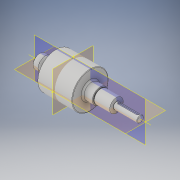
# Autodesk Inventor part: vratilo
Saved by Autodesk Inventor 2018 (Build 220112000, 112)
## iProperties
Created: 2018-05-05
Part Number: vratilo
Material: Generic
Document SubType Name: Modeling
Designer: Kristijan
Density: 1 g/cm^3
Appearance: Default
Author: Kristijan
Autodesk Inventor part; units mm, degrees
sketch "Sketch1" plane through (0, 0, 0) normal (1, 0, 0) x (0, 1, 0)
  circle A0 centre (0, 0) radius 60.5
  dimension "d0" = 121
  constraints: 1 centre point, 1 coincident
  measures "d0" diameter of A0
extrude "Extrusion1" add sketch "Sketch1" along normal mid plane 115
sketch "Sketch2" plane through (57.5, 0, 0) normal (1, 0, 0) x (0, 0, -1)
  circle A0 centre (0, 0) radius 26
  dimension "d3" = 52
  constraints: 1 centre point, 1 coincident
  measures "d3" diameter of A0
extrude "Extrusion2" add sketch "Sketch2" along normal blind 33
sketch "Sketch3" plane through (90.5, 0, 0) normal (1, 0, 0) x (0, 0, -1)
  circle A0 centre (0, 0) radius 22.5
  dimension "d6" = 45
  constraints: 1 centre point, 1 coincident
  measures "d6" diameter of A0
extrude "Extrusion3" add sketch "Sketch3" along normal blind 54
sketch "Sketch4" plane through (144.5, 0, 0) normal (1, 0, 0) x (0, 0, -1)
  circle A0 centre (0, 0) radius 11
  dimension "d9" = 22
  constraints: 1 centre point, 1 coincident
  measures "d9" diameter of A0
extrude "Extrusion4" add sketch "Sketch4" along normal blind 80
mirror "Mirror1" about plane through (0, 0, 0) normal (1, 0, 0) of "Extrusion2"
sketch "Sketch5" plane through (-90.5, 0, 0) normal (-1, 0, 0) x (0, 0, 1)
  circle A0 centre (0, 0) radius 22.5
  dimension "d12" = 45
  constraints: 1 centre point, 1 coincident
  measures "d12" diameter of A0
extrude "Extrusion5" add sketch "Sketch5" along normal blind 21
ref_plane "Work Plane1" through (144.5, 0, 11) normal (0, 0, 1) x (1, 0, 0)
sketch "Sketch6" plane through (144.5, 0, 11) normal (0, 0, 1) x (1, 0, 0)
  line L0 (9, 0) -> (71, 0) construction
  line L1 (9, -4) -> (71, -4)
  line L2 (71, 4) -> (9, 4)
  arc A0 (9, 4) -> (9, -4) centre (9, 0) ccw
  arc A1 (71, -4) -> (71, 4) centre (71, 0) ccw
  line L3 (80, -11) -> (80, 11) construction
  line L4 (-258.4, 0) -> (136.4, 0) construction
  line L5 (0, -22.5) -> (0, 22.5) construction
  point P0 (-144.5, 0)
  point P1 (40, 0)
  dimension "d15" = 62
  dimension "d16" = 8
  dimension "d18" = 5
  constraints: 8 end point, 4 point on circle, 4 tangent, 2 centre point, 1 collinear, 1 horizontal, 1 midpoint, 1 parallel
  measures "d15" distance of L0.start L0.end
  measures "d16" diameter of A1
  measures "d18" distance edge to line of A1 L3
extrude "Extrusion6" cut sketch "Sketch6" against normal blind 5
sketch "Sketch7" plane through (0, 0, 0) normal (0, 1, 0) x (-1, 0, 0)
  line L0 (-57.5, -26) -> (-90.5, -26) construction
  line L1 (-90.5, -26) -> (-90.5, -22.5) construction
  line L2 (-90.5, -22.5) -> (-144.5, -22.5) construction
  line L3 (-144.5, -22.5) -> (-144.5, -11) construction
  line L4 (-144.5, -11) -> (-224.5, -11) construction
  line L5 (-224.5, -11) -> (-224.5, 11) construction
  line L6 (-224.5, 11) -> (-219.5, 11) construction
  line L7 (-219.5, 11) -> (-219.5, 6) construction
  line L8 (-219.5, 6) -> (-149.5, 6) construction
  line L9 (-149.5, 6) -> (-149.5, 11) construction
  line L10 (-149.5, 11) -> (-144.5, 11) construction
  line L11 (-144.5, 11) -> (-144.5, 22.5) construction
  line L12 (-144.5, 22.5) -> (-90.5, 22.5) construction
  line L13 (-90.5, 22.5) -> (-90.5, 26) construction
  line L14 (-90.5, 26) -> (-57.5, 26) construction
  line L15 (-57.5, 26) -> (-57.5, 60.5) construction
  line L16 (-57.5, 60.5) -> (57.5, 60.5) construction
  line L17 (57.5, 60.5) -> (57.5, 26) construction
  line L18 (57.5, 26) -> (90.5, 26) construction
  line L19 (90.5, 26) -> (90.5, 22.5) construction
  line L20 (90.5, 22.5) -> (111.5, 22.5) construction
  line L21 (111.5, 22.5) -> (111.5, -22.5) construction
  line L22 (111.5, -22.5) -> (90.5, -22.5) construction
  line L23 (90.5, -22.5) -> (90.5, -26) construction
  line L24 (90.5, -26) -> (57.5, -26) construction
  line L25 (57.5, -26) -> (57.5, -60.5) construction
  line L26 (57.5, -60.5) -> (-57.5, -60.5) construction
  line L27 (-57.5, -60.5) -> (-57.5, -26) construction
  line L28 (-93, 15.4374) -> (-93, 22.5) construction
  line L29 (-90.5, 22.5) -> (-144.5, 22.5) construction
  line L30 (-93, 22.5) -> (-90.5, 22.5)
  line L31 (-90.5, 22.2) -> (-91.8804, 22.2)
  line L32 (-90.5, 26) -> (-90.5, -26) construction
  line L33 (-93, 22.5) -> (-91.8804, 22.2)
  line L34 (-90.5, 22.5) -> (-93, 22.5) construction
  line L35 (-90.5, 22.5) -> (-90.5, 22.2)
  line L36 (125.9, 0) -> (-198.9, 0) projected
  point P0 (0, 0)
  dimension "d21" = 2.5
  dimension "d24" = 0.3
  dimension "d25" = 15
  constraints: 12 end point, 3 point on line, 2 collinear, 2 horizontal, 1 vertical
  measures "d21" distance between parallel lines of L28 L13
  measures "d24" distance between parallel lines of L12 L31
  measures "d25" angle of L12 L33
revolve "Revolution1" cut sketch "Sketch7" angle 360 about axis through (-10, 0, 0) along (1, 0, 0)
mirror "Mirror2" about plane through (0, 0, 0) normal (1, 0, 0) of "Revolution1"
fillet "Fillet1" radius 0.6 1 edges at (90.5, 0, -22.2)
fillet "Fillet2" radius 0.6 1 edges at (91.8804, 0, -22.2)
fillet "Fillet3" radius 0.6 1 edges at (-90.5, 0, -22.2)
fillet "Fillet4" radius 0.6 1 edges at (-91.8804, 0, -22.2)
fillet "Fillet5" radius 0.6 1 edges at (144.5, 0, 11)
fillet "Fillet6" radius 5 2 edges at (57.5, 0, 26) (-57.5, 0, 26)
chamfer "Chamfer1" distance 1.5 angle 45 2 edges at (-111.5, 0, -22.5) (224.5, 0, 11)
chamfer "Chamfer2" distance 2 angle 30 1 edges at (57.5, -60.5, 0) measured on face at (57.5, -60, 0)
chamfer "Chamfer3" distance 2 angle 30 1 edges at (-57.5, -60.5, 0) measured on face at (-57.5, -60, 0)
body "Solid1"
